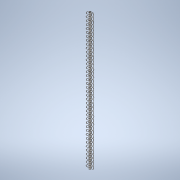
# Autodesk Inventor part: marble_lift_shaft
Saved by Autodesk Inventor 2020 (Build 240168000, 168)
## iProperties
Created: 2021-03-06
Part Number: marble_lift_shaft
Material: Generic
Document SubType Name: Modeling
Designer: Harry
Density: 1 g/cm^3
Appearance: Knurled 45
Author: Harry
Autodesk Inventor part; units mm, degrees
ref_plane "YZ Plane" through (0, 0, 0) normal (1, 0, 0) x (0, 1, 0)
ref_plane "XZ Plane" through (0, 0, 0) normal (0, 1, 0) x (-1, 0, 0)
ref_plane "XY Plane" through (0, 0, 0) normal (0, 0, 1) x (1, 0, 0)
sketch "Sketch1" plane through (0, 0, 0) normal (0, 1, 0) x (-1, 0, 0)
  circle A0 centre (0, 0) radius 5
  dimension "d0" = 10
  constraints: 1 centre point, 1 coincident
  measures "d0" diameter of A0
extrude "Extrusion1" add sketch "Sketch1" along normal blind 800
sketch "Sketch2" plane through (0, 0, 0) normal (0, 0, 1) x (1, 0, 0)
  circle A0 centre (5.6962, 2.9579) radius 1
  line L0 (5.6962, 2.9579) -> (15.6962, 2.9579) construction
  circle A1 centre (15.6962, 2.9579) radius 1
  point P0 (0, 0)
  dimension "d3" = 2
  dimension "d4" = 10
  dimension "d5" = 2
  constraints: 2 centre point, 2 end point, 1 coincident, 1 horizontal
  measures "d3" diameter of A0
  measures "d4" distance of L0.start L0.end
  measures "d5" diameter of A1
coil "Coil1" sketch "Sketch2" operation add axis through (0, -10, 0) along (0, 1, 0) pitch 20 turns 40 hand right
sketch "Sketch3" plane through (0, 0, 0) normal (0, 0, 1) x (1, 0, 0)
  arc A0 (6.6962, 2.9579) -> (5, 3.6758) centre (5.6962, 2.9579) ccw projected
  circle A1 centre (15.6962, 2.9579) radius 1 projected
  line L0 (5.6962, 2.9579) -> (15.6962, 2.9579) construction
  line L1 (6.6962, 1.9579) -> (14.6962, 1.9579)
  line L2 (14.6962, 3.9579) -> (6.6962, 3.9579)
  arc A2 (6.6962, 3.9579) -> (6.6962, 1.9579) centre (6.6962, 2.9579) ccw
  arc A3 (14.6962, 1.9579) -> (14.6962, 3.9579) centre (14.6962, 2.9579) ccw
  point P0 (0, 0)
  point P1 (16.6962, 2.9579)
  point P2 (10.6962, 2.9579)
  point P3 (15.1962, 2.0919)
  point P4 (15.1962, 3.824)
  constraints: 8 end point, 6 point on circle, 4 tangent, 2 centre point, 2 point on line, 1 horizontal, 1 midpoint, 1 parallel
extrude "Extrusion2" [suppressed]
pattern_linear "Rectangular Pattern1" [suppressed]
body "Solid1"
